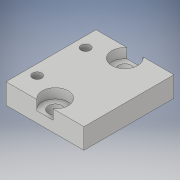
# Autodesk Inventor part: LidarV4MountShortPlate
Saved by Autodesk Inventor 2019 (Build 230136000, 136)
## iProperties
Created: 2020-08-15
Part Number: LidarV4MountShortPlate
Material: Generic
Document SubType Name: Modeling
Designer: james
Density: 1 g/cm^3
Appearance: Default
Author: james
Autodesk Inventor part; units mm, degrees
ref_plane "YZ Plane" through (0, 0, 0) normal (1, 0, 0) x (0, 1, 0)
ref_plane "XZ Plane" through (0, 0, 0) normal (0, 1, 0) x (-1, 0, 0)
ref_plane "XY Plane" through (0, 0, 0) normal (0, 0, 1) x (1, 0, 0)
sketch "Sketch1" plane through (0, 0, 0) normal (1, 0, 0) x (0, 1, 0)
  line L0 (1.2948, 31.3833) -> (-8.7052, 31.3833)
  line L1 (-8.7052, 31.3833) -> (-8.7052, -12.6095)
  line L2 (-8.7052, -12.6095) -> (1.2948, -12.6095)
  line L3 (1.2948, -12.6095) -> (1.2948, 31.3833)
  point P0 (0, 0)
  dimension "d0" = 43.9928
  dimension "d1" = 10
  constraints: 8 end point, 2 parallel, 1 horizontal, 1 perpendicular
  measures "d0" distance of L0.end L1.end
  measures "d1" distance of L0.start L0.end
extrude "Extrusion1" add sketch "Sketch1" along normal blind 38.1
sketch "Sketch2" plane through (0, 1.2948, 31.3833) normal (0, 1, 0) x (1, 0, 0)
  line L0 (38.1, 43.9928) -> (38.1, 0) projected
  line L1 (0, 0) -> (38.1, 0) projected
  line L2 (0, 43.9928) -> (38.1, 43.9928) projected
  point P0 (0, 31.3833)
  point P1 (19.05, 5)
  point P2 (19.05, 38.9928)
  dimension "d4" = 0
  dimension "d5" = 19.05
  dimension "d6" = 5
  dimension "d7" = 5
  measures "d4" horizontal distance of point (19.05, 5) point (19.05, 38.993)
  measures "d5" distance from line of L0 point (19.05, 5)
  measures "d6" distance from line of L1 point (19.05, 5)
  measures "d7" distance from line of L2 point (19.05, 38.993)
hole "Hole1" at (19.05, 1.2948, 26.3833) at (19.05, 1.2948, -7.6095) direction (0, -1, 0) diameter 6.7564 end through all counterbore diameter 12.7 counterbore depth 4.7752 clearance for "Hex Head Bolt" size "1/4" standard "Ansi Unified Screw Threads"
sketch "Sketch3" plane through (0, -8.7052, -12.6095) normal (0, -1, 0) x (1, 0, 0)
  line L0 (38.1, 43.9928) -> (38.1, 0) projected
  line L1 (0, 43.9928) -> (0, 0) projected
  line L2 (0, 43.9928) -> (38.1, 43.9928) projected
  line L3 (0, 0) -> (38.1, 0) projected
  point P0 (0, 12.6095)
  point P1 (5.08, 33.8328)
  point P2 (5.08, 10.16)
  dimension "d16" = 5.08
  dimension "d24" = 10.16
  dimension "d25" = 10.16
  dimension "d26" = 5.08
  measures "d16" distance from line of L1 point (5.08, 10.16)
  measures "d24" distance from line of L2 point (5.08, 33.833)
  measures "d25" distance from line of L3 point (5.08, 10.16)
  measures "d26" distance from line of point (5.08, 33.833) L1
hole "Hole2" at (5.08, -8.7052, 21.2233) at (5.08, -8.7052, -2.4495) direction (0, 1, 0) diameter 4.4958 end through all clearance for "Hex Machine Screw" size "#8" standard "Ansi Unified Screw Threads"
body "Solid1"
